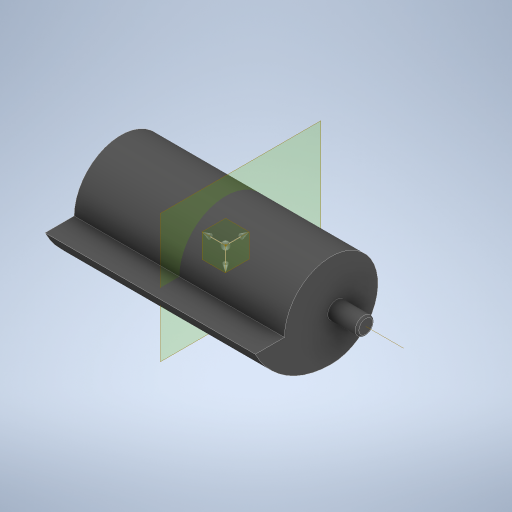
# Autodesk Inventor part: Drum
Saved by Autodesk Inventor 2024 (Build 280153000, 153)
## iProperties
Created: 2023-10-18
Part Number: Drum
Material: Generic
Document SubType Name: Modeling
Designer: CJ110
Density: 1 g/cm^3
Appearance: Default
Mass: 194.247 g
Surface Area: 207.239 cm^2
Volume: 194.247 cm^3
Author: CJ110
## iProperties of the stored document Drum_3DPrint.ipt
Created: 2023-11-07
Part Number: Drum_3DPrint
Material: Generic
Document SubType Name: Modeling
Designer: CJ110
Density: 1 g/cm^3
Appearance: Default
Author: CJ110
Autodesk Inventor part; units mm, degrees
ref_plane "YZ Plane" through (0, 0, 0) normal (1, 0, 0) x (0, 1, 0)
ref_plane "XZ Plane" through (0, 0, 0) normal (0, 1, 0) x (-1, 0, 0)
ref_plane "XY Plane" through (0, 0, 0) normal (0, 0, 1) x (1, 0, 0)
sketch "Sketch1" plane through (0, 0, 0) normal (0, 1, 0) x (-1, 0, 0)
  circle A0 centre (0, 0) radius 20.32
  line L0 (0, 0) -> (0, 20.32) construction
  line L1 (0, 0) -> (-20.32, 0) construction
  line L2 (0, 20.32) -> (0, -20.32) construction
  line L3 (0, -20.32) -> (0, -33.02)
  arc A1 (-20.32, 0) -> (0, -33.02) centre (16.6688, 0) ccw
  point P0 (0, 20.32)
  dimension "d0" = 40.64
  dimension "d12" = 12.7
  constraints: 8 end point, 6 point on circle, 3 vertical, 2 centre point, 1 coincident, 1 horizontal, 1 tangent
  measures "d0" diameter of A0
  measures "d12" distance of L2.end L3.end
extrude "Extrusion1" add sketch "Sketch1" along normal blind 91.44
ref_plane "Work Plane1" through (0, 45.72, 0) normal (0, 1, 0) x (1, 0, 0)
sketch "Sketch2" plane through (0, 91.44, 0) normal (0, 1, 0) x (1, 0, 0)
  circle A0 centre (0.8355, -2.3151) radius 2.921
  circle A1 centre (0.8355, -2.3151) radius 3.81
  circle A2 centre (0.8355, -2.3151) radius 2.286
  point P0 (0, 0)
  dimension "d5" = 5.842
  dimension "d6" = 7.62
  dimension "d11" = 4.572
  constraints: 3 centre point, 2 coincident
  measures "d5" diameter of A0
  measures "d6" diameter of A1
  measures "d11" diameter of A2
extrude "Extrusion2" add sketch "Sketch2" against normal blind 12.7 from surface at -91.44 contours A0 | A1 | A2
extrude "Extrusion3" cut sketch "Sketch2" against normal blind 13.97 contours A0 | A2
fillet "Fillet1" radius 0.7937 1 edges at (-2.9745, -12.7, 2.3151)
body "Solid1"
